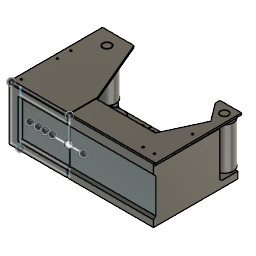
SpoolmanScale_test_model (Autodesk Fusion 360 design; units mm, degrees)
Autodesk Fusion 360 part; units mm, degrees
note: some values were not read from the file. Chosen so that the rebuilt part matches the saved one: which face or edge a step refers to. Set by a fixed rule: which sketch regions a step uses.
sketch "Szkic1" plane through (0, 0, 0) normal (0, 0, 1) x (1, 0, 0)
  circle A0 centre (0, 0) radius 100
  circle A1 centre (0, -120) radius 20
  line L0 (-100, 0) -> (-110, 0)
  line L1 (100, 0) -> (110, 0)
  circle A2 centre (-130, 0) radius 20
  circle A3 centre (130, 0) radius 20
  circle A4 centre (130, 0) radius 10
  circle A5 centre (0, -120) radius 10
  circle A6 centre (-130, 0) radius 10
  dimension "d1" = 200
  dimension "d5" = 20
  constraint coincident A0.centre origin
  constraint tangent A0 A1
  constraint coincident A0 L0.start
  constraint horizontal L0
  constraint coincident A0 L1.start
  constraint horizontal L1
  constraint coincident L0.end A2
  constraint coincident L1.end A3
  constraint concentric A3 A4
  constraint concentric A1 A5
  constraint concentric A2 A6
  measures "d1" diameter of A0
  measures "d5" diameter of A4
extrude "Wyciągnięcie proste1" add sketch "Szkic1" along normal blind 78 contours A1 | A2 | A3 | A4 | A5 | A6 makes body 1 at (149.9751, -0.9969, 26) makes body 2 at (19.9006, -118.0086, 52) makes body 3 at (-110.0249, -0.9969, 52)
extrude "Wyciągnięcie proste2" cut sketch "Szkic1" along normal blind 80 contours A4 | A5 | A6 bodies 1 2 3
sketch "Szkic2" plane through (0, 0, 0) normal (0, 0, 1) x (1, 0, 0)
  circle A0 centre (130, 0) radius 8.5
  circle A1 centre (-130, 0) radius 8.5
  circle A2 centre (0, -120) radius 8.5
  line L0 (0, -145) -> (9.525, -145)
  line L1 (0, -145) -> (-9.525, -145)
  line L2 (-9.525, -145) -> (-9.525, -150)
  line L3 (9.525, -145) -> (9.525, -150)
  line L4 (9.525, -150) -> (-9.525, -150)
  line L5 (9.525, -145) -> (25.525, -145)
  line L6 (25.525, -145) -> (8.5, -120)
  line L7 (-9.525, -145) -> (-25.525, -145)
  line L8 (-25.525, -145) -> (-8.5, -120)
  line L9 (-25.525, -145) -> (-25.525, -150)
  line L10 (-25.525, -150) -> (-9.525, -150)
  line L11 (25.525, -145) -> (25.525, -150)
  line L12 (25.525, -150) -> (9.525, -150)
  circle A3 centre (0, -120) radius 25
  dimension "d8" = 17
  dimension "d9" = 17
  dimension "d10" = 17
  dimension "d19" = 9.525
  dimension "d20" = 9.525
  dimension "d21" = 16
  dimension "d22" = 16
  constraint horizontal L0
  constraint parallel L0 L1
  constraint perpendicular L1 L2
  constraint perpendicular L0 L3
  constraint perpendicular L2 L4
  constraint perpendicular L3 L5
  constraint coincident A2 L6.end
  constraint perpendicular L2 L7
  constraint coincident A2 L8.end
  constraint perpendicular L7 L9
  constraint perpendicular L2 L10
  constraint perpendicular L5 L11
  constraint perpendicular L3 L12
  constraint concentric A2 A3
  constraint coincident L0.start A3
  constraint tangent L1 A3
  measures "d8" diameter of A0
  measures "d9" diameter of A1
  measures "d10" diameter of A2
  measures "d19" distance of L0.start L0.end
  measures "d20" distance of L0.start L1.end
  measures "d21" distance of L0.end L5.end
  measures "d22" distance of L1.end L7.end
extrude "Wyciągnięcie proste3" add sketch "Szkic2" along normal blind 90 separate body contours A0 | A1 | A2 makes body 4 at (8.4578, -120.8463, 30) makes body 5 at (138.4894, -0.4237, 60) makes body 6 at (-121.5106, -0.4237, 60)
extrude "Wyciągnięcie proste4" add sketch "Szkic2" against normal blind 10 contours A2 L6 L8 A3 | A2 L6 L8 A3 | L0 L5 L6 A3 | L1 L7 L8 A3 | L3 L5 L11 L12 | L0 L1 L2 L3 L4 | L2 L7 L9 L10 bodies 4
extrude "Wyciągnięcie proste5" add 1 faces at (-0.2117, -142.8254, 0) along direction (0, 0, 1) blind 10 from surface at 80 separate body on bodies 4 makes body 7
sketch "Szkic4" plane through (0, 0, 90) normal (0, 0, 1) x (-1, 0, 0)
  circle A0 centre (0, 120) radius 8.5
  line L0 (-25.525, 145) -> (-19.3117, 135.8763)
  arc A1 (-19.3117, 135.8763) -> (19.3117, 135.8763) centre (0, 120) ccw
  line L1 (19.3117, 135.8763) -> (25.525, 145)
  line L2 (25.525, 145) -> (25.525, 150)
  line L3 (25.525, 150) -> (-25.525, 150)
  line L4 (-25.525, 150) -> (-25.525, 145)
  circle A2 centre (0, 120) radius 8.5
  circle A3 centre (0, 120) radius 9.1
  dimension "d29" = 18.2
  constraint tangent A0 A2
  constraint concentric A2 A3
  measures "d29" diameter of A3
extrude "Wyciągnięcie proste6" cut sketch "Szkic4" against normal blind 10 contours A0 A2 | A3 bodies 7
sketch "Szkic6" plane through (0, -150, 0) normal (0, -1, 0) x (1, 0, 0)
  line L0 (25.525, 0) -> (-25.525, 0)
  line L1 (-25.525, 0) -> (-25.525, -10)
  line L2 (-25.525, -10) -> (25.525, -10)
  line L3 (25.525, -10) -> (25.525, 0)
  line L4 (30, 90) -> (-25.525, 90)
  line L5 (-25.525, 90) -> (-25.525, -10)
  line L6 (-25.525, -10) -> (30, -10)
  line L7 (30, -10) -> (30, 90)
  line L8 (-25.525, -10) -> (30, -10)
  line L9 (30, -10) -> (30, -15)
  line L10 (30, -15) -> (-25.525, -15)
  line L11 (-25.525, -15) -> (-25.525, -10)
  line L12 (30, 90) -> (-25.525, 90)
  line L13 (-25.525, 90) -> (-25.525, 95.054)
  line L14 (-25.525, 95.054) -> (30, 95.054)
  line L15 (30, 95.054) -> (30, 90)
  line L16 (-25.525, 95.054) -> (-30, 95.054)
  line L17 (-30, 95.054) -> (-30, -15)
  line L18 (-30, -15) -> (-25.525, -15)
  line L19 (-25.525, -15) -> (-25.525, 95.054)
  line L20 (30, 95.054) -> (30, 40.027)
  line L21 (30, 40.027) -> (-30, 40.027)
  line L22 (0, 40.027) -> (9.525, 40.027)
  line L23 (0, 40.027) -> (-9.525, 40.027)
  circle A0 centre (9.525, 40.027) radius 2.7
  circle A1 centre (-9.525, 40.027) radius 2.7
  dimension "d32" = 55.027
  dimension "d33" = 9.525
  dimension "d34" = 9.525
  dimension "d35" = 5.4
  dimension "d36" = 5.4
  constraint horizontal L4
  constraint vertical L5
  constraint horizontal L6
  constraint vertical L7
  constraint coincident L1.end L2.start
  constraint horizontal L8
  constraint vertical L9
  constraint horizontal L10
  constraint vertical L11
  constraint horizontal L12
  constraint vertical L13
  constraint horizontal L14
  constraint vertical L15
  constraint horizontal L16
  constraint vertical L17
  constraint horizontal L18
  constraint vertical L19
  constraint perpendicular L10 L20
  constraint midpoint L17 L21.end
  constraint midpoint L21 L22.start
  constraint perpendicular L7 L22
  constraint parallel L21 L23
  constraint coincident L22.end A0.centre
  constraint coincident L23.end A1.centre
  measures "d32" distance of L14.end L20.end
  measures "d33" distance of L22.start L22.end
  measures "d34" distance of L22.start L23.end
  measures "d35" diameter of A0
  measures "d36" diameter of A1
extrude "Wyciągnięcie proste7" add sketch "Szkic6" along normal blind 10 and the other way blind 0 contours L0 L1 L2 L3 L5 L6 L8 L19 | L0 L3 L5 L6 L7 L8 L19 L21 L22 L23 A0 A1 | L1 L5 L11 L17 L18 L19 L21 | L2 L6 L8 L9 L10 L11 L19 | L5 L13 L16 L17 L19 L21 | L4 L5 L7 L12 L19 L20 L21 L22 L23 A0 A1 | L4 L12 L13 L14 L15 L19 L20 bodies 4
extrude "Wyciągnięcie proste8" add 1 faces at (0.2117, -142.8254, -10) along direction (0, 0, -1) blind 5 on bodies 4 bodies 4
extrude "Wyciągnięcie proste9" add 1 faces at (2.133, -120.216, 0) along direction (0, 0, -1) blind 15 on bodies 4 bodies 4
fillet "Zaokrąglenie1" radius 5 2 edges at (-25.525, -150, -7.5) (25.525, -150, -7.5) on bodies 4
fillet "Zaokrąglenie2" radius 5 2 edges at (-19.3117, -135.8763, -7.5) (19.3117, -135.8763, -7.5) on bodies 4
extrude "Wyciągnięcie proste10" add 2 faces at (-127.3214, -2.0645, 0) (131.8924, 3.0503, 0) along direction (0, 0, -1) blind 15 on bodies 5 6 bodies 6 5
sketch "Szkic7" plane through (0, 0, -15) normal (0, 0, -1) x (1, 0, 0)
  line L0 (-25.525, 145.0276) -> (-25.525, 145)
  line L1 (-25.525, 145) -> (-21.2772, 138.7624)
  arc A0 (-21.1749, 133.29) -> (-21.2772, 138.7624) centre (-25.4099, 135.948) ccw
  arc A1 (-21.1749, 133.29) -> (21.1749, 133.29) centre (0, 120) ccw
  arc A2 (21.2772, 138.7624) -> (21.1749, 133.29) centre (25.4099, 135.948) ccw
  line L2 (21.2772, 138.7624) -> (25.525, 145)
  line L3 (25.525, 145) -> (25.525, 145.0276)
  arc A3 (30, 150) -> (25.525, 145.0276) centre (30.525, 145.0276) ccw
  line L4 (30, 150) -> (30, 160)
  line L5 (30, 160) -> (-30, 160)
  line L6 (-30, 160) -> (-30, 150)
  arc A4 (-25.525, 145.0276) -> (-30, 150) centre (-30.525, 145.0276) ccw
  line L7 (150, -10) -> (-40, -10)
  line L8 (-40, -10) -> (-40, 170)
  line L9 (-40, 170) -> (150, 170)
  line L10 (150, 170) -> (150, -10)
  line L11 (-41, -10) -> (-170, -10)
  line L12 (-170, -10) -> (-170, 170)
  line L13 (-170, 170) -> (-41, 170)
  line L14 (-41, 170) -> (-41, -10)
  line L15 (150, 30) -> (130, 30)
  line L16 (130, 30) -> (70, 160)
  line L17 (-170, 10) -> (-150, 20)
  line L18 (-30, 160) -> (-110, 160)
  line L19 (-110, 160) -> (-110, 170)
  line L20 (-30, 170) -> (-30, 160)
  line L21 (150, 170) -> (150, 172)
  line L22 (-170, 172) -> (-170, 170)
  line L23 (-150, 20) -> (-150, 170)
  line L24 (70, 160) -> (70, 170)
  line L25 (-40, 170) -> (-40, 172)
  line L26 (-41, 172) -> (-41, 170)
  line L27 (-110, 170) -> (-41, 170)
  line L28 (-40, 170) -> (-30, 170)
  line L29 (150, 172) -> (-40, 172)
  line L30 (-41, 172) -> (-170, 172)
  dimension "d51" = 1
  dimension "d60" = 80
  dimension "d61" = 2
  constraint horizontal L7
  constraint vertical L8
  constraint horizontal L9
  constraint vertical L10
  constraint horizontal L11
  constraint vertical L12
  constraint horizontal L13
  constraint vertical L14
  constraint coincident L10 L15.start
  constraint perpendicular L10 L15
  constraint coincident L12 L17.start
  constraint horizontal L18
  constraint vertical L19
  constraint horizontal L27
  constraint vertical L20
  constraint coincident L5.end L6.start
  constraint perpendicular L9 L21
  constraint perpendicular L10 L29
  constraint perpendicular L13 L22
  constraint coincident L13 L23.end
  constraint perpendicular L13 L23
  constraint coincident L9 L24.end
  constraint perpendicular L9 L24
  constraint vertical L25
  constraint vertical L26
  constraint collinear L27 L28
  constraint collinear L29 L30
  measures "d51" distance of L7.end L11.start
  measures "d60" distance of L5.end L18.end
  measures "d61" distance of L9.end L21.end
extrude "Wyciągnięcie proste13" add sketch "Szkic7" along normal blind 5 contours L11 L12 L13 L14 L17 L18 L19 L23 | L13 L14 L18 L19 L27 | L12 L13 L17 L23 bodies 6
extrude "Wyciągnięcie proste14" add sketch "Szkic7" along normal blind 5 contours L0 L1 A0 A1 A2 L2 L3 A3 L4 L5 L6 A4 | L7 L8 L9 L10 L15 L16 L18 L20 L24 | L8 L9 L18 L20 L28 | L9 L10 L15 L16 L24 bodies 5
extrude "Wyciągnięcie proste15" add sketch "Szkic7" along normal blind 5 contours L9 L21 L25 L28 L29 | L13 L22 L26 L27 L30 bodies 6 5
extrude "Wyciągnięcie proste16" add sketch "Szkic7" against normal blind 112 contours L9 L21 L25 L28 L29 | L9 L10 L15 L16 L24 | L12 L13 L17 L23 | L13 L22 L26 L27 L30 bodies 6 5
sketch "Szkic8" plane through (0, 0, -15) normal (0, 0, -1) x (1, 0, 0)
  line L0 (-35.0805, 0.0384) -> (-45, 0.0384)
  line L1 (-45, 0.0384) -> (-53, 0.0384)
  line L2 (-56.6, -2.04) -> (-53, -4.1185)
  line L3 (-53, -4.1185) -> (-49.4, -2.04)
  line L4 (-49.4, -2.04) -> (-49.4, 2.1169)
  line L5 (-49.4, 2.1169) -> (-53, 4.1954)
  line L6 (-53, 4.1954) -> (-56.6, 2.1169)
  line L7 (-56.6, 2.1169) -> (-56.6, -2.04)
  line L8 (-35.0805, 0.0384) -> (-30, 0)
  line L9 (-26.4109, 2.0972) -> (-30.0217, 4.1569)
  line L10 (-30.0217, 4.1569) -> (-33.6108, 2.0597)
  line L11 (-33.6108, 2.0597) -> (-33.5891, -2.0972)
  line L12 (-33.5891, -2.0972) -> (-29.9783, -4.1569)
  line L13 (-29.9783, -4.1569) -> (-26.3892, -2.0597)
  line L14 (-26.3892, -2.0597) -> (-26.4109, 2.0972)
  line L15 (-18.6, 87.9215) -> (-15, 85.8431)
  line L16 (-15, 85.8431) -> (-11.4, 87.9215)
  line L17 (-11.4, 87.9215) -> (-11.4, 92.0785)
  line L18 (-11.4, 92.0785) -> (-15, 94.1569)
  line L19 (-15, 94.1569) -> (-18.6, 92.0785)
  line L20 (-18.6, 92.0785) -> (-18.6, 87.9215)
  line L21 (-58.6, 87.9215) -> (-55, 85.8431)
  line L22 (-55, 85.8431) -> (-51.4, 87.9215)
  line L23 (-51.4, 87.9215) -> (-51.4, 92.0785)
  line L24 (-51.4, 92.0785) -> (-55, 94.1569)
  line L25 (-55, 94.1569) -> (-58.6, 92.0785)
  line L26 (-58.6, 92.0785) -> (-58.6, 87.9215)
  line L27 (0, 100) -> (-80, 100)
  line L28 (-80, 100) -> (-80, -10)
  line L29 (-80, -10) -> (0, -10)
  line L30 (0, -10) -> (0, 100)
  circle A0 centre (-15, 90) radius 2.15
  circle A1 centre (-55, 90) radius 2.15
  circle A2 centre (-53, 0.0384) radius 2.15
  circle A3 centre (-30, 0) radius 2.15
  point P0 (-30, 0)
  point P1 (-53, 0.0384)
  point P2 (-30, 0)
  point P3 (-15, 90)
  point P4 (-55, 90)
  dimension "d67" = 3.6
  dimension "d68" = 3.6
  dimension "d69" = 3.6
  dimension "d70" = 3.6
  dimension "d71" = 4.3
  dimension "d72" = 4.3
  dimension "d73" = 4.3
  dimension "d74" = 4.3
  constraint horizontal L0
  constraint parallel L0 L1
  constraint coincident P1 L1.end
  constraint coincident P0 L8.end
  constraint horizontal L27
  constraint vertical L28
  constraint horizontal L29
  constraint vertical L30
  constraint coincident P3 A0.centre
  constraint coincident P4 A1.centre
  measures "d67" distance of P1 L7
  measures "d68" distance of P2 L14
  measures "d69" distance of P3 L20
  measures "d70" distance of P4 L26
  measures "d71" diameter of A0
  measures "d72" diameter of A1
  measures "d73" diameter of A2
  measures "d74" diameter of A3
extrude "Wyciągnięcie proste17" add sketch "Szkic8" along normal blind 3 from surface at 5 separate body contours L2 L3 L4 L5 L6 L7 | L9 L10 L11 L12 L13 L14 | L15 L16 L17 L18 L19 L20 | L21 L22 L23 L24 L25 L26 | L27 L28 L29 L30 makes body 8
extrude "Wyciągnięcie proste18" cut sketch "Szkic8" along normal blind 2 contours L2 L3 L4 L5 L6 L7 | L9 L10 L11 L12 L13 L14 | L15 L16 L17 L18 L19 L20 | L21 L22 L23 L24 L25 L26 | A0 | A1 | A2 | A3 bodies 6 5
extrude "Wyciągnięcie proste19" cut sketch "Szkic8" along normal blind 10 contours A0 | A1 | A2 | A3 bodies 6 5
sketch "Szkic9" plane through (0, 0, -15) normal (0, 0, 1) x (-1, 0, 0)
  line L0 (29.9783, -4.1569) -> (26.3892, -2.0597)
  line L1 (26.3892, -2.0597) -> (26.4109, 2.0972)
  line L2 (26.4109, 2.0972) -> (30.0217, 4.1569)
  line L3 (30.0217, 4.1569) -> (33.6108, 2.0597)
  line L4 (33.6108, 2.0597) -> (33.5891, -2.0972)
  line L5 (33.5891, -2.0972) -> (29.9783, -4.1569)
  line L6 (15, 94.1569) -> (18.6, 92.0785)
  line L7 (18.6, 92.0785) -> (18.6, 87.9215)
  line L8 (18.6, 87.9215) -> (15, 85.8431)
  line L9 (15, 85.8431) -> (11.4, 87.9215)
  line L10 (11.4, 87.9215) -> (11.4, 92.0785)
  line L11 (11.4, 92.0785) -> (15, 94.1569)
  circle A0 centre (-130, 0) radius 8.5
  line L12 (40, 170) -> (-70, 170)
  line L13 (-70, 170) -> (-70, 160)
  line L14 (-70, 160) -> (-130, 30)
  line L15 (-130, 30) -> (-150, 30)
  line L16 (-150, 30) -> (-150, -10)
  line L17 (-150, -10) -> (40, -10)
  line L18 (40, -10) -> (40, 170)
  line L19 (-130, 30) -> (-100, -10)
  line L20 (-150, -10) -> (-150, 30)
  line L21 (-130, 30) -> (-150, 30)
  line L22 (-150, -10) -> (-100, -10)
  constraint coincident L14.end L15.start
  constraint coincident L17 L19.end
  constraint coincident L16.end L17.start
  constraint coincident L15.end L16.start
extrude "Wyciągnięcie proste20" add sketch "Szkic9" along normal blind 10 contours L15 L16 L17 L19 L20 L21 L22 bodies 5
chamfer "Fazowanie1" distance 4 angle 45 1 edges at (140, -30, -5) on bodies 5
chamfer "Fazowanie2" distance 3 angle 45 1 edges at (115, -10, -15) on bodies 5
chamfer "Fazowanie3" distance 3 angle 45 1 edges at (99.2857, -96.5476, -15) on bodies 5
sketch "Szkic10" plane through (0, 0, -15) normal (0, 0, 1) x (-1, 0, 0)
  line L0 (53, 4.1954) -> (56.6, 2.1169)
  line L1 (56.6, 2.1169) -> (56.6, -2.04)
  line L2 (56.6, -2.04) -> (53, -4.1185)
  line L3 (53, -4.1185) -> (49.4, -2.04)
  line L4 (49.4, -2.04) -> (49.4, 2.1169)
  line L5 (49.4, 2.1169) -> (53, 4.1954)
  line L6 (55, 94.1569) -> (58.6, 92.0785)
  line L7 (58.6, 92.0785) -> (58.6, 87.9215)
  line L8 (58.6, 87.9215) -> (55, 85.8431)
  line L9 (55, 85.8431) -> (51.4, 87.9215)
  line L10 (51.4, 87.9215) -> (51.4, 92.0785)
  line L11 (51.4, 92.0785) -> (55, 94.1569)
  line L12 (150, 170) -> (41, 170)
  line L13 (41, 170) -> (41, -10)
  line L14 (41, -10) -> (170, -10)
  line L15 (170, -10) -> (170, 10)
  line L16 (170, 10) -> (150, 20)
  line L17 (150, 20) -> (150, 170)
  circle A0 centre (130, 0) radius 8.5
  line L18 (115, -10) -> (115, 10)
  line L19 (115, 10) -> (150, 20)
  line L20 (170, 10) -> (150, 20)
  line L21 (170, 10) -> (170, -10)
  line L22 (170, -10) -> (115, -10)
  constraint coincident L14 L18.start
  constraint perpendicular L14 L18
  constraint coincident L16.end L17.start
  constraint coincident L15.end L16.start
  constraint coincident L14.end L15.start
extrude "Wyciągnięcie proste21" add sketch "Szkic10" along normal blind 10 contours L14 L15 L16 L18 L19 L20 L21 L22 bodies 6
chamfer "Fazowanie4" distance 3 angle 45 4 edges at (-160, -15, -5) (-132.5, -15, -15) (-150, -95, -15) (-115, 0, -15) on bodies 6
sketch "Szkic11" plane through (0, 0, 97) normal (0, 0, 1) x (-1, 0, 0)
  line L0 (-150, 172) -> (-150, 30)
  line L1 (-150, 30) -> (-130, 30)
  line L2 (-130, 30) -> (-70, 160)
  line L3 (-70, 160) -> (-70, 170)
  line L4 (-70, 170) -> (40, 170)
  line L5 (40, 170) -> (40, 172)
  line L6 (40, 172) -> (-150, 172)
  line L7 (-130, 30) -> (-100, -10)
  line L8 (-148.4615, -10) -> (-150, 172)
  line L9 (-150, 172) -> (-149.9998, 172)
  line L10 (40, 170) -> (40, 172)
  line L11 (40, 172) -> (-149.9998, 172)
  line L12 (-91.1312, 114.2158) -> (-130, 30)
  circle A0 centre (-130, 0) radius 8.9
  line L13 (-91.1312, 114.2158) -> (40, 114.2158)
  line L14 (40, 114.2158) -> (40, 170)
  line L15 (-100, -10) -> (-100, -20)
  line L16 (-100, -20) -> (-148.4615, -20)
  line L17 (-148.4615, -20) -> (-148.4615, -10)
  line L18 (-133.6, 152.9215) -> (-130, 150.8431)
  line L19 (-130, 150.8431) -> (-126.4, 152.9215)
  line L20 (-126.4, 152.9215) -> (-126.4, 157.0785)
  line L21 (-126.4, 157.0785) -> (-130, 159.1569)
  line L22 (-130, 159.1569) -> (-133.6, 157.0785)
  line L23 (-133.6, 157.0785) -> (-133.6, 152.9215)
  line L24 (-108.6988, 154.9071) -> (-106.769, 151.7503)
  line L25 (-106.769, 151.7503) -> (-103.0701, 151.8432)
  line L26 (-103.0701, 151.8432) -> (-101.3012, 155.0929)
  line L27 (-101.3012, 155.0929) -> (-103.2311, 158.2497)
  line L28 (-103.2311, 158.2497) -> (-106.9299, 158.1568)
  line L29 (-106.9299, 158.1568) -> (-108.6988, 154.9071)
  line L30 (-131.3, 75) -> (-133.15, 78.2043)
  line L31 (-133.15, 78.2043) -> (-136.85, 78.2043)
  line L32 (-136.85, 78.2043) -> (-138.7, 75)
  line L33 (-138.7, 75) -> (-136.85, 71.7957)
  line L34 (-136.85, 71.7957) -> (-133.15, 71.7957)
  line L35 (-133.15, 71.7957) -> (-131.3, 75)
  circle A1 centre (-135, 75) radius 2.15
  circle A2 centre (-130, 155) radius 2.15
  circle A3 centre (-105, 155) radius 2.15
  point P0 (-130, 155)
  point P1 (-105, 155)
  point P2 (-135, 75)
  dimension "d90" = 17.8
  dimension "d91" = 3.6
  dimension "d92" = 3.7
  dimension "d93" = 3.7
  dimension "d94" = 4.3
  dimension "d95" = 4.3
  dimension "d96" = 4.3
  constraint coincident L1.end L2.start
  constraint coincident L0.start L6.end
  constraint perpendicular L8 L9
  constraint coincident L5.end L6.start
  constraint horizontal L13
  constraint vertical L14
  constraint coincident L4.end L5.start
  constraint perpendicular L15 L16
  constraint coincident P2 A1.centre
  constraint coincident P0 A2.centre
  constraint coincident P1 A3.centre
  measures "d90" diameter of A0
  measures "d91" distance of P0 L23
  measures "d92" distance of L24.start P1
  measures "d93" distance of L30.start P2
  measures "d94" diameter of A1
  measures "d95" diameter of A2
  measures "d96" diameter of A3
extrude "Wyciągnięcie proste22" cut sketch "Szkic11" against normal blind 5 from surface at -10 contours L18 L19 L20 L21 L22 L23 | L24 L25 L26 L27 L28 L29 | L30 L31 L32 L33 L34 L35 | A1 | A2 | A3 bodies 5
extrude "Wyciągnięcie proste23" cut sketch "Szkic11" against normal blind 20 contours A1 | A2 | A3 bodies 5
extrude "Wyciągnięcie proste24" add sketch "Szkic11" along normal blind 4 separate body contours L1 L2 L3 L4 L5 L6 L8 L10 L11 L12 | L1 L7 L8 L15 L16 L17 | L2 L3 L4 L13 L14 | L18 L19 L20 L21 L22 L23 | L24 L25 L26 L27 L28 L29 | L30 L31 L32 L33 L34 L35 makes body 9
sketch "Szkic12" plane through (0, 0, 97) normal (0, 0, 1) x (-1, 0, 0)
  line L0 (150, 20) -> (170, 10)
  line L1 (170, 10) -> (170, 172)
  line L2 (170, 172) -> (41, 172)
  line L3 (41, 172) -> (41, 170)
  line L4 (41, 170) -> (150, 170)
  line L5 (150, 170) -> (150, 20)
  line L6 (170, 10) -> (170, -10)
  line L7 (170, -10) -> (170, -30)
  line L8 (170, -30) -> (100, -30)
  line L9 (100, -30) -> (41, 110)
  line L10 (41, 110) -> (41, 172)
  line L11 (41, 172) -> (170, 172)
  line L12 (170, 172) -> (170, 10)
  circle A0 centre (130, 0) radius 9.5
  line L13 (156.3, 47.8638) -> (160, 45.7276)
  line L14 (160, 45.7276) -> (163.7, 47.8638)
  line L15 (163.7, 47.8638) -> (163.7, 52.1362)
  line L16 (163.7, 52.1362) -> (160, 54.2724)
  line L17 (160, 54.2724) -> (156.3, 52.1362)
  line L18 (156.3, 52.1362) -> (156.3, 47.8638)
  line L19 (156.3, 157.8638) -> (160, 155.7276)
  line L20 (160, 155.7276) -> (163.7, 157.8638)
  line L21 (163.7, 157.8638) -> (163.7, 162.1362)
  line L22 (163.7, 162.1362) -> (160, 164.2724)
  line L23 (160, 164.2724) -> (156.3, 162.1362)
  line L24 (156.3, 162.1362) -> (156.3, 157.8638)
  line L25 (156.3524, 77.7754) -> (160.1028, 75.7288)
  line L26 (160.1028, 75.7288) -> (163.7503, 77.9534)
  line L27 (163.7503, 77.9534) -> (163.6476, 82.2246)
  line L28 (163.6476, 82.2246) -> (159.8972, 84.2712)
  line L29 (159.8972, 84.2712) -> (156.2497, 82.0466)
  line L30 (156.2497, 82.0466) -> (156.3524, 77.7754)
  circle A1 centre (160, 80) radius 2.15
  circle A2 centre (160, 50) radius 2.15
  circle A3 centre (160, 160) radius 2.15
  line L31 (41, 172) -> (170, 172)
  line L32 (170, 172) -> (170, 171)
  line L33 (170, 171) -> (41, 171)
  line L34 (41, 171) -> (41, 172)
  line L35 (170, 172) -> (40.9434, 172)
  line L36 (40.9434, 172) -> (40.9434, 176)
  line L37 (40.9434, 176) -> (170, 176)
  line L38 (170, 176) -> (170, 172)
  point P0 (160, 50)
  point P1 (160, 160)
  point P2 (160, 80)
  dimension "d104" = 19
  dimension "d105" = 3.7
  dimension "d106" = 3.7
  dimension "d107" = 3.7
  dimension "d108" = 4.3
  dimension "d109" = 4.3
  dimension "d110" = 4.3
  dimension "d138" = 1
  dimension "d139" = 4
  constraint coincident L0.end L1.start
  constraint parallel L1 L6
  constraint parallel L1 L7
  constraint perpendicular L7 L8
  constraint coincident L2.end L3.start
  constraint coincident L1.end L2.start
  constraint coincident P2 A1.centre
  constraint coincident P0 A2.centre
  constraint coincident P1 A3.centre
  constraint horizontal L31
  constraint vertical L32
  constraint horizontal L33
  constraint vertical L34
  constraint coincident L12 L32.end
  constraint horizontal L35
  constraint vertical L36
  constraint horizontal L37
  constraint vertical L38
  measures "d104" diameter of A0
  measures "d105" distance of P0 L18
  measures "d106" distance of P1 L24
  measures "d107" distance of P2 L30
  measures "d108" diameter of A1
  measures "d109" diameter of A2
  measures "d110" diameter of A3
  measures "d138" distance of L2.end L33.end
  measures "d139" distance of L1.end L37.end
extrude "Wyciągnięcie proste25" add 1 faces at (-127.3214, -2.0645, 90) along direction (0, 0, 1) blind 11 on bodies 6 bodies 6
extrude "Wyciągnięcie proste26" add 1 faces at (131.8924, 3.0503, 90) along direction (0, 0, 1) blind 11 on bodies 5 bodies 5
extrude "Wyciągnięcie proste27" cut sketch "Szkic12" against normal blind 5 from surface at -5 contours L13 L14 L15 L16 L17 L18 | L19 L20 L21 L22 L23 L24 | L25 L26 L27 L28 L29 L30 | A1 | A2 | A3 bodies 6
extrude "Wyciągnięcie proste28" cut sketch "Szkic12" against normal blind 20 contours A1 | A2 | A3 bodies 6
extrude "Wyciągnięcie proste29" add sketch "Szkic12" along normal blind 4 separate body contours L0 L1 L3 L4 L5 L10 L12 L33 | L0 L4 L5 L6 L7 L8 L9 L10 | L1 L2 L3 L10 L11 L12 L31 L32 L33 L34 L35 | L13 L14 L15 L16 L17 L18 | L19 L20 L21 L22 L23 L24 | L25 L26 L27 L28 L29 L30 makes body 10
sketch "Szkic13" plane through (0, -172, 0) normal (0, -1, 0) x (1, 0, 0)
  line L0 (-170, 97) -> (-170, -20)
  line L1 (-170, -20) -> (-41, -20)
  line L2 (-41, -20) -> (-41, 97)
  line L3 (-41, 97) -> (-170, 97)
  line L4 (-41, 97) -> (-41, 42)
  circle A0 centre (-9.5248, 39.991) radius 2.72
  line L5 (-9.5248, 39.991) -> (-109.5248, 39.991)
  line L6 (-109.5248, 39.991) -> (-128.5748, 39.991)
  line L7 (-109.5248, 39.991) -> (-109.5248, 41.991)
  line L8 (-128.5748, 39.991) -> (-128.5748, 41.991)
  circle A1 centre (-109.5248, 41.991) radius 2.65
  circle A2 centre (-128.5748, 41.991) radius 2.65
  line L9 (-109.5248, 41.991) -> (-95, 41.991)
  circle A3 centre (-95, 41.991) radius 2.65
  line L10 (-128.5058, 44.6401) -> (-95.0001, 44.641)
  line L11 (-128.5747, 39.341) -> (-95, 39.341)
  circle A4 centre (-79, 41.991) radius 2.65
  line L12 (-95.0001, 44.641) -> (-79, 44.641)
  line L13 (-79, 39.341) -> (-95, 39.341)
  line L14 (-95, 41.991) -> (-92.35, 41.991)
  line L15 (-81.65, 41.991) -> (-79, 41.991)
  line L16 (-170, 97) -> (-150, 97)
  line L17 (-150, 97) -> (-150, -20)
  line L18 (-150, -20) -> (-170, -20)
  line L19 (-170, -20) -> (-170, 97)
  line L20 (-150, 97) -> (-41, 97)
  line L21 (-41, 97) -> (-41, 82)
  line L22 (-41, 82) -> (-150, 82)
  line L23 (-150, 82) -> (-150, 97)
  line L24 (-150, -20) -> (-41, -20)
  line L25 (-41, -20) -> (-41, -5)
  line L26 (-41, -5) -> (-150, -5)
  line L27 (-150, -5) -> (-150, -20)
  dimension "d122" = 55
  dimension "d123" = 100
  dimension "d124" = 19.05
  dimension "d127" = 2
  dimension "d128" = 2
  dimension "d129" = 5.3
  dimension "d130" = 5.3
  dimension "d131" = 5.3
  dimension "d132" = 5.3
  dimension "d133" = 15
  dimension "d134" = 15
  constraint coincident L2.end L3.start
  constraint perpendicular L3 L4
  constraint coincident A0.centre L5.start
  constraint perpendicular L2 L5
  constraint perpendicular L2 L6
  constraint perpendicular L6 L7
  constraint perpendicular L6 L8
  constraint coincident L7.end A1.centre
  constraint coincident L8.end A2.centre
  constraint perpendicular L7 L9
  constraint coincident L9.end A3.centre
  constraint coincident A2 L10.start
  constraint coincident A3 L10.end
  constraint tangent A3 L10
  constraint coincident A2 L11.start
  constraint coincident A3 L11.end
  constraint tangent A3 L11
  constraint parallel L9 L14
  constraint coincident A4.centre L15.end
  constraint coincident A4 L12.end
  constraint tangent A4 L12
  constraint coincident A4 L13.start
  constraint tangent A3 L13
  constraint coincident A3 L14.end
  constraint coincident A4 L15.start
  constraint collinear L14 L15
  constraint horizontal L16
  constraint vertical L17
  constraint horizontal L18
  constraint vertical L19
  constraint coincident L1 L17.end
  constraint coincident L0.start L3.end
  constraint horizontal L20
  constraint vertical L21
  constraint horizontal L22
  constraint vertical L23
  constraint horizontal L24
  constraint vertical L25
  constraint horizontal L26
  constraint vertical L27
  measures "d122" distance of L2.end L4.end
  measures "d123" distance of A0.centre L5.end
  measures "d124" distance of L5.end L6.end
  measures "d127" distance of L5.end L7.end
  measures "d128" distance of L6.end L8.end
  measures "d129" diameter of A1
  measures "d130" diameter of A2
  measures "d131" diameter of A3
  measures "d132" diameter of A4
  measures "d133" distance of L16.end L22.end
  measures "d134" distance of L17.end L26.end
extrude "Wyciągnięcie proste30" add sketch "Szkic13" along normal blind 5 contours L0 L1 L3 L16 L17 L18 L19 L23 L27 | L2 L3 L4 L17 L20 L21 L22 L23 | L1 L2 L17 L24 L25 L26 L27 bodies 6
chamfer "Fazowanie5" distance 5 angle 45 3 edges at (-95.5, -172, -5) (-150, -172, 38.5) (-95.5, -172, 82) on bodies 6
sketch "Szkic15" plane through (0, -172, 0) normal (0, -1, 0) x (1, 0, 0)
  line L0 (-40, 97) -> (-40, -20)
  line L1 (-40, -20) -> (150, -20)
  line L2 (150, -20) -> (150, 97)
  line L3 (150, 97) -> (-40, 97)
extrude "Wyciągnięcie proste31" add sketch "Szkic12" along normal blind 4 contours L2 L11 L31 L35 L36 L37 L38 bodies 6
chamfer "Fazowanie6" distance 1 angle 45 1 edges at (-105.5, -176, 97) on bodies 6
sketch "Szkic16" plane through (0, -172, 0) normal (0, -1, 0) x (1, 0, 0)
  line L0 (-40, -20) -> (150, -20)
  line L1 (150, -20) -> (150, -5)
  line L2 (150, -5) -> (-40, -5)
  line L3 (-40, -5) -> (-40, -20)
  line L4 (-40, 97) -> (150, 97)
  line L5 (150, 97) -> (150, 82)
  line L6 (150, 82) -> (-40, 82)
  line L7 (-40, 82) -> (-40, 97)
  dimension "d143" = 190
  dimension "d144" = 15
  dimension "d145" = 190
  dimension "d146" = 15
  constraint horizontal L0
  constraint vertical L1
  constraint horizontal L2
  constraint vertical L3
  constraint horizontal L4
  constraint vertical L5
  constraint horizontal L6
  constraint vertical L7
  measures "d143" distance of L0.start L0.end
  measures "d144" distance of L0.start L2.end
  measures "d145" distance of L4.start L4.end
  measures "d146" distance of L4.start L6.end
extrude "Wyciągnięcie proste32" add sketch "Szkic16" along normal blind 5 bodies 5
chamfer "Fazowanie7" distance 5 angle 45 2 edges at (55, -172, -5) (55, -172, 82) on bodies 5
extrude "Wyciągnięcie proste33" add 1 faces at (-113.445, -1.4904, 78) along direction (0, 0, 1) blind 15 on bodies 3 bodies 3
extrude "Wyciągnięcie proste34" add 1 faces at (146.555, 1.4904, 78) along direction (0, 0, 1) blind 15 on bodies 1 bodies 1
sketch "Szkic17" plane through (0, 0, 97) normal (0, 0, 1) x (-1, 0, 0)
  circle A0 centre (-130, 155) radius 2.15
  circle A1 centre (-105, 155) radius 2.15
  circle A2 centre (-135, 75) radius 2.15
  line L0 (-150, 172) -> (-150, 30)
  line L1 (-150, 30) -> (-130, 30)
  line L2 (-130, 30) -> (-70, 160)
  line L3 (-70, 160) -> (-70, 170)
  line L4 (-70, 170) -> (40, 170)
  line L5 (40, 170) -> (40, 177)
  line L6 (40, 177) -> (-150, 177)
  line L7 (-150, 177) -> (-150, 172)
  line L8 (40, 177) -> (-149.8935, 177)
  line L9 (-149.8935, 177) -> (-149.8935, 173)
  line L10 (-149.8935, 173) -> (40, 173)
  line L11 (40, 173) -> (40, 177)
  dimension "d154" = 4
  constraint horizontal L8
  constraint vertical L9
  constraint horizontal L10
  constraint vertical L11
  constraint coincident L5.end L6.start
  measures "d154" distance of L5.end L10.end
extrude "Wyciągnięcie proste35" add sketch "Szkic17" along normal blind 5 contours L5 L6 L8 L9 L10 L11 bodies 5
extrude "Wyciągnięcie proste36" cut sketch "Szkic13" against normal blind 10 contours L5 A4 | L5 A4 | L5 A3 A4 L13 | L5 A3 A4 L12 | L5 A3 | L5 L9 A3 L14 | L5 A1 A3 L11 | L5 A1 L9 A3 | L9 A3 L14 | L6 A1 A2 L11 | L5 L6 A1 | A1 L9 A3 L10 | L5 L7 A1 L9 | L6 L7 A1 L9 | L6 A1 A2 L10 | A2 bodies 6
equation "d19 = ( 19.05 / 2 ) * 1 mm"
equation "d20 = ( 19.05 / 2 ) * 1 mm"
equation "d32 = 110.054 mm - ( ( 110.054 / 2 ) * 1 mm )"
equation "d33 = ( 19.05 / 2 ) * 1 mm"
equation "d34 = ( 19.05 / 2 ) * 1 mm"
equation "d67 = ( 7.2 / 2 ) * 1 mm"
equation "d68 = ( 7.2 / 2 ) * 1 mm"
equation "d69 = ( 7.2 / 2 ) * 1 mm"
equation "d70 = ( 7.2 / 2 ) * 1 mm"
equation "d91 = ( 7.2 / 2 ) * 1 mm"
equation "d92 = ( 7.4 / 2 ) * 1 mm"
equation "d93 = ( 7.4 / 2 ) * 1 mm"
equation "d105 = ( 7.4 / 2 ) * 1 mm"
equation "d106 = ( 7.4 / 2 ) * 1 mm"
equation "d107 = ( 7.4 / 2 ) * 1 mm"
equation "d122 = ( 110 / 2 ) * 1 mm"
named bodies: "tensor_roller", "tenso_pala_all", "right_part", "left_part", "tenso_pala_upper", "plate", "cover_right", "left_cover"
